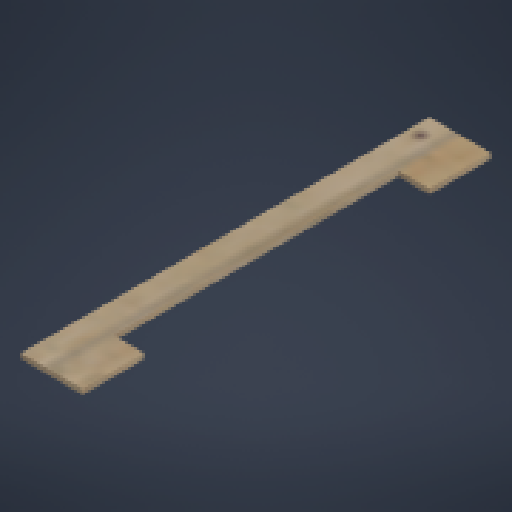
# Autodesk Inventor part: belt_rail
Saved by Autodesk Inventor 2026.1 (Build 301233020, 233B)
## iProperties
Created: 2025-09-28
Part Number: belt_rail
Material: 木材 (カエデ材)
Document SubType Name: Modeling
Designer: hibik
Density: 0.67 g/cm^3
Appearance: ナチュラル カエデ材 - 光沢 濃い着色
Author: hibik
Autodesk Inventor part; units mm, degrees
ref_plane "YZ Plane" through (0, 0, 0) normal (1, 0, 0) x (0, 1, 0)
ref_plane "XZ Plane" through (0, 0, 0) normal (0, 1, 0) x (-1, 0, 0)
ref_plane "XY Plane" through (0, 0, 0) normal (0, 0, 1) x (1, 0, 0)
sketch "スケッチ1" plane through (0, 0, 0) normal (0, 1, 0) x (-1, 0, 0)
  line L0 (0, 99) -> (30, 99)
  line L1 (30, 99) -> (30, -99)
  line L2 (30, -99) -> (0, -99)
  line L3 (0, -99) -> (0, 99)
  line L4 (0, -69) -> (15, -69)
  line L5 (15, -69) -> (15, 0)
  line L6 (36, 0) -> (-6, 0) projected
  line L7 (0, 69) -> (15, 69)
  line L8 (15, 69) -> (15, 0)
  point P0 (0, 0)
  point P1 (0, 0)
  dimension "d0" = 198
  dimension "d1" = 30
  dimension "d32" = 30
  dimension "d33" = 15
  constraints: 16 end point, 3 perpendicular, 2 parallel, 2 symmetric about line, 1 coincident, 1 horizontal, 1 horizontal alignment, 1 midpoint, 1 point on line
  measures "d0" distance of L0.end L1.end
  measures "d1" distance of L0.start L0.end
  measures "d32" distance between parallel lines of L2 L4
  measures "d33" distance between parallel lines of L3 L5
extrude "押し出し1" add sketch "スケッチ1" along normal blind 2.5 contours L0 L1 L6 L8 L7 L3 | L1 L2 L3 L4 L5 L6
